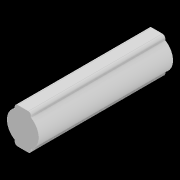
# Autodesk Inventor part: Axel_parametriserad_02
Saved by Autodesk Inventor 2020 (Build 240168000, 168)
## iProperties
Created: 2020-11-21
Part Number: Axel_parametriserad_02
Material: Generic
Document SubType Name: Modeling
Designer: Gottfrid
Density: 1 g/cm^3
Appearance: Default
Author: Gottfrid
Autodesk Inventor part; units mm, degrees
ref_plane "YZ Plane" through (0, 0, 0) normal (1, 0, 0) x (0, 1, 0)
ref_plane "XZ Plane" through (0, 0, 0) normal (0, 1, 0) x (-1, 0, 0)
ref_plane "XY Plane" through (0, 0, 0) normal (0, 0, 1) x (1, 0, 0)
sketch "Sketch1" plane through (0, 0, 0) normal (0, 0, 1) x (1, 0, 0)
  circle A0 centre (0, 0) radius 2.95
  line L0 (1, -3.3333) -> (-1, -3.3333)
  line L1 (-1.5, -2.8333) -> (-1.5, 2.8333)
  line L2 (-1, 3.3333) -> (1, 3.3333)
  line L3 (1.5, 2.8333) -> (1.5, -2.8333)
  line L4 (1.5, -3.3333) -> (-1.5, 3.3333) construction
  line L5 (-1.5, -3.3333) -> (1.5, 3.3333) construction
  arc A1 (-1, 3.3333) -> (-1.5, 2.8333) centre (-1, 2.8333) ccw
  arc A2 (1.5, 2.8333) -> (1, 3.3333) centre (1, 2.8333) ccw
  arc A3 (1, -3.3333) -> (1.5, -2.8333) centre (1, -2.8333) ccw
  arc A4 (-1.5, -2.8333) -> (-1, -3.3333) centre (-1, -2.8333) ccw
  point P0 (-1.5, 3.3333)
  point P1 (-1.5, 3.3333)
  point P2 (1.5, 3.3333)
  point P3 (1.5, 3.3333)
  point P4 (1.5, 3.3333)
  point P5 (1.5, -3.3333)
  point P6 (-1.5, -3.3333)
  point P7 (-1.5, -3.3333)
  point P8 (-1.5, -3.3333)
  point P9 (1.5, 2.5402)
  point P10 (-1.5, 2.5402)
  point P11 (-1.5, -2.5402)
  point P12 (1.5, -2.5402)
  point P13 (-1.5, 3.3333)
  point P14 (1.5, 3.3333)
  point P15 (1.5, 3.3333)
  point P16 (1.5, 3.3333)
  point P17 (1.5, -3.3333)
  point P18 (-1.5, -3.3333)
  point P19 (-1.5, -3.3333)
  point P20 (-1.5, -3.3333)
  dimension "d0" = 5.9
  dimension "d1" = 6.6667
  dimension "d2" = 3
  dimension "d7" = 0.5
  constraints: 24 point on line, 12 end point, 9 horizontal, 8 point on circle, 8 tangent, 8 vertical, 5 centre point, 3 equal radius, 2 midpoint, 2 parallel, 1 coincident, 1 perpendicular, 32 other
  measures "d0" diameter of A0
  measures "d1" distance between parallel lines of L0 L2
  measures "d2" distance between parallel lines of L3 L1
  measures "d7" radius of A1
extrude "Extrusion1" add sketch "Sketch1" along normal blind 25
equation "\"d0\" = D_axel - d_toleransAxel"
equation "\"d7\" = r_filletAxel"
equation "\"d4\" = h_axel"
equation "\"d_toleransAxel\" = 0.1"
equation "\"d_inreRing_fromMagneticRotor\" = 2"
equation "\"h_axel\" = 25"
equation "\"r_filletAxel\" = 0.5"
equation "\"D_axel\" = 6"
body "Solid1"
